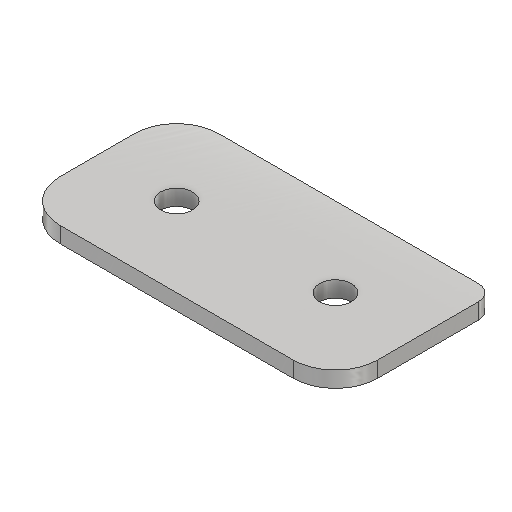
# Autodesk Inventor part: LC_ALU_3mm_30x30_Rectangular_Bracket
Saved by Autodesk Inventor 2026.1 (Build 301233000, 233)
## iProperties
Created: 2016-06-27
Part Number: LC_ALU_3mm_30x30_Rectangular_Bracket
Material: Ogólny
Document SubType Name: Modeling
Designer: Andrzej
Density: 1 g/cm^3
Appearance: Obrobione — aluminium
Author: Andrzej
Autodesk Inventor part; units mm, degrees
ref_plane "YZ Plane" through (0, 0, 0) normal (1, 0, 0) x (0, 1, 0)
ref_plane "XZ Plane" through (0, 0, 0) normal (0, 1, 0) x (-1, 0, 0)
ref_plane "XY Plane" through (0, 0, 0) normal (0, 0, 1) x (1, 0, 0)
sketch "Szkic1" plane through (0, 0, 0) normal (0, 0, 1) x (1, 0, 0)
  line L0 (-57.3371, 37.8455) -> (-57.3371, 7.8455)
  line L1 (-57.3371, 7.8455) -> (2.6629, 7.8455)
  line L2 (2.6629, 7.8455) -> (2.6629, 37.8455)
  line L3 (2.6629, 37.8455) -> (-57.3371, 37.8455)
  point P0 (0, 0)
  point P1 (-42.3371, 22.8455)
  point P2 (-12.3371, 22.8455)
  dimension "d0" = 30
  dimension "d2" = 60
  dimension "d4" = 15
  dimension "d6" = 15
  dimension "d7" = 15
  dimension "d9" = 15
  constraints: 8 end point, 2 perpendicular, 1 vertical
  measures "d0" distance of L0.start L0.end
  measures "d2" distance of L1.end L0.end
  measures "d4" distance from line of L3 point (-42.337, 22.846)
  measures "d6" distance from line of L3 point (-12.337, 22.846)
  measures "d7" distance from line of L2 point (-12.337, 22.846)
  measures "d9" distance from line of point (-42.337, 22.846) L0
extrude "Wyciągnięcie proste1" add sketch "Szkic1" along normal blind 3
hole "Otwór1" at (-42.3371, 22.8455, 0) at (-12.3371, 22.8455, 0) direction (0, 0, 1) diameter 6 end through all
fillet "Zaokrąglenie2" radius 3 1 edges at (2.6629, 37.8455, 1.5)
fillet "Zaokrąglenie3" radius 8 3 edges at (2.6629, 7.8455, 1.5) (-57.3371, 7.8455, 1.5) (-57.3371, 37.8455, 1.5)
equation "\"d4\" = 0.5 * d0"
equation "\"d6\" = d5"
equation "\"d7\" = d5"
equation "\"d5\" = 0.5 * d1"
equation "\"d1\" = 30"
